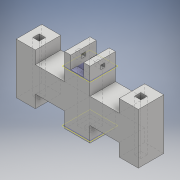
# Autodesk Inventor part: PRING_piston
Saved by Autodesk Inventor 2018 (Build 220112000, 112)
## iProperties
Created: 2026-07-07
Part Number: PRING_piston
Material: Generic
Document SubType Name: Modeling
Designer: neo
Density: 1 g/cm^3
Appearance: Default
Author: neo
Autodesk Inventor part; units mm, degrees
ref_plane "YZ Plane" through (0, 0, 0) normal (1, 0, 0) x (0, 1, 0)
ref_plane "XZ Plane" through (0, 0, 0) normal (0, 1, 0) x (-1, 0, 0)
ref_plane "XY Plane" through (0, 0, 0) normal (0, 0, 1) x (1, 0, 0)
sketch "Sketch1" plane through (0, 0, 0) normal (0, 1, 0) x (-1, 0, 0)
  line L0 (41.98, 54.6032) -> (41.98, -104.2857) construction
  line L1 (-38.02, 54.6032) -> (-38.02, -101.9048) construction
  line L2 (49.98, -31.1313) -> (-46.02, -31.1313)
  line L3 (-46.02, -31.1313) -> (-46.02, -71.1313)
  line L4 (-46.02, -71.1313) -> (49.98, -71.1313)
  line L5 (49.98, -71.1313) -> (49.98, -31.1313)
  line L6 (1.98, 80.3555) -> (1.98, -108.9591)
  point P0 (0, 0)
  dimension "d0" = 80
  dimension "d1" = 8
  dimension "d2" = 40
  constraints: 14 end point, 3 vertical, 2 parallel, 1 horizontal, 1 perpendicular, 2 other
  measures "d0" distance between parallel lines of L1 L0
  measures "d1" distance between parallel lines of L0 L5
  measures "d2" distance of L4.end L2.start
extrude "Extrusion1" add sketch "Sketch1" along normal mid plane 20
sketch "Sketch2" plane through (46.02, 10, -71.1313) normal (0, 0, -1) x (-1, 0, 0)
  circle A0 centre (88, -10) radius 2.5 construction
  circle A1 centre (8, -10) radius 2.5 construction
  line L0 (10.5, -7.5) -> (5.5, -7.5)
  line L1 (5.5, -7.5) -> (5.5, -12.5)
  line L2 (5.5, -12.5) -> (10.5, -12.5)
  line L3 (10.5, -12.5) -> (10.5, -7.5)
  line L4 (85.5, -7.5) -> (90.5, -7.5)
  line L5 (90.5, -7.5) -> (90.5, -12.5)
  line L6 (90.5, -12.5) -> (85.5, -12.5)
  line L7 (85.5, -12.5) -> (85.5, -7.5)
  point P0 (46.02, -10)
  point P1 (88, -10)
  point P2 (8, -10)
  dimension "d5" = 5
  dimension "d6" = 5
  constraints: 16 end point, 8 tangent, 4 parallel, 2 centre point, 2 coincident, 2 horizontal, 2 perpendicular
  measures "d5" diameter of A0
  measures "d6" diameter of A1
extrude "Extrusion2" cut sketch "Sketch2" against normal through all
sketch "Sketch3" plane through (0, 10, 0) normal (0, 1, 0) x (1, 0, 0)
  line L0 (-49.98, 31.1313) -> (46.02, 31.1313) construction
  line L1 (46.02, 31.1313) -> (46.02, 71.1313) construction
  line L2 (46.02, 71.1313) -> (-49.98, 71.1313) construction
  line L3 (-49.98, 71.1313) -> (-49.98, 31.1313) construction
  line L4 (-34.98, 79.1313) -> (31.02, 79.1313)
  line L5 (31.02, 79.1313) -> (31.02, 61.1313)
  line L6 (31.02, 61.1313) -> (-34.98, 61.1313)
  line L7 (-34.98, 61.1313) -> (-34.98, 79.1313)
  line L8 (46.02, 31.1313) -> (-49.98, 31.1313) construction
  line L9 (-1.98, 31.1313) -> (-1.98, 128.9069) construction
  line L10 (-41.98, -54.6032) -> (-41.98, 104.2857) construction
  line L11 (-34.98, 23.1313) -> (31.02, 23.1313)
  line L12 (31.02, 23.1313) -> (31.02, 41.1313)
  line L13 (31.02, 41.1313) -> (-34.98, 41.1313)
  line L14 (-34.98, 41.1313) -> (-34.98, 23.1313)
  point P0 (0, 0)
  dimension "d9" = 7
  dimension "d10" = 10
  dimension "d11" = 18
  dimension "d14" = 10
  dimension "d15" = 18
  constraints: 18 end point, 4 parallel, 2 horizontal, 2 perpendicular, 1 collinear, 1 midpoint, 1 vertical, 2 other
  measures "d9" distance between parallel lines of L10 L7
  measures "d10" distance between parallel lines of L6 L2
  measures "d11" distance of L6.end L4.start
  measures "d14" distance between parallel lines of L13 L8
  measures "d15" distance of L13.end L11.start
extrude "Extrusion3" cut sketch "Sketch3" against normal through all
sketch "Sketch4" plane through (31.02, 10, -61.1313) normal (0, 0, -1) x (-1, 0, 0)
  line L0 (31.02, -10) -> (61.64, -10) construction
  line L1 (43, 0) -> (23, 0)
  line L2 (23, 0) -> (23, -20)
  line L3 (23, -20) -> (43, -20)
  line L4 (43, -20) -> (43, 0)
  line L5 (66, -20) -> (0, -20) construction
  line L6 (66, 0) -> (66, -20) construction
  line L7 (0, 0) -> (66, 0) construction
  line L8 (0, 0) -> (0, -20) construction
  line L9 (66, -20) -> (0, -20) construction
  line L10 (33, -20) -> (33, -66.7058) construction
  line L11 (66, -10) -> (82.2472, -10) construction
  dimension "d16" = 20
  constraints: 14 end point, 2 midpoint, 2 parallel, 2 perpendicular, 1 collinear, 1 vertical, 2 other
  measures "d16" distance of L1.start L1.end
extrude "Extrusion4" add sketch "Sketch4" along normal blind 12 and the other way blind 40.5
ref_plane "Work Plane1" through (31.02, 10, -71.1313) normal (0, 0, -1) x (-1, 0, 0)
sketch "Sketch5" plane through (31.02, 10, -71.1313) normal (0, 0, -1) x (-1, 0, 0)
  line L0 (43, 0) -> (23, 0) construction
  line L1 (23, 0) -> (23, -20) construction
  line L2 (23, -20) -> (43, -20) construction
  line L3 (43, -20) -> (43, 0) construction
  line L4 (38.1, -4.9) -> (27.9, -4.9)
  line L5 (27.9, -4.9) -> (27.9, -15.1)
  line L6 (27.9, -15.1) -> (38.1, -15.1)
  line L7 (38.1, -15.1) -> (38.1, -4.9)
  line L8 (43, 0) -> (23, 0) construction
  line L9 (33, 0) -> (33, -20) construction
  line L10 (43, -20) -> (43, 0) construction
  line L11 (43, -10) -> (23, -10) construction
  line L12 (23, 0) -> (23, -20) construction
  point P0 (31.02, -10)
  dimension "d28" = 10.2
  constraints: 12 end point, 4 midpoint, 2 parallel, 2 perpendicular, 1 horizontal, 2 other
  measures "d28" distance of L6.end L4.start
extrude "Extrusion5" cut sketch "Sketch5" against normal through all
ref_plane "Work Plane2" through (31.02, 10, -30.6313) normal (0, 0, -1) x (-1, 0, 0)
sketch "Sketch6" plane through (31.02, 10, -20.6313) normal (0, 0, 1) x (1, 0, 0)
  line L0 (-38.1, -25.1) -> (-27.9, -25.1)
  line L1 (-27.9, -25.1) -> (-27.9, 5.1)
  line L2 (-27.9, 5.1) -> (-38.1, 5.1)
  line L3 (-38.1, 5.1) -> (-38.1, -25.1)
  line L4 (-38.1, -4.9) -> (-27.9, -4.9) construction
  line L5 (-38.1, -15.1) -> (-38.1, -4.9) construction
  line L6 (-27.9, -15.1) -> (-38.1, -15.1) construction
  line L7 (-27.9, -4.9) -> (-27.9, -15.1) construction
  line L8 (-38.1, -15.1) -> (-38.1, -4.9) construction
  line L9 (-27.9, -4.9) -> (-27.9, -15.1) construction
  point P0 (-31.02, -10)
  dimension "d29" = 10
  dimension "d30" = 10
  constraints: 8 end point, 2 collinear, 2 parallel, 1 horizontal, 1 perpendicular
  measures "d29" distance between parallel lines of L0 L6
  measures "d30" distance between parallel lines of L2 L4
extrude "Extrusion6" cut sketch "Sketch6" against normal up to surface (10 mm away)
sketch "Sketch7" plane through (-11.98, -10, -41.1313) normal (-1, 0, 0) x (0, 0, 1)
  line L0 (10.5, -4) -> (10.5, 24) construction
  line L1 (0, 0) -> (0, 20) construction
  line L2 (20.5, 0) -> (0, 0) construction
  line L3 (20.5, 20) -> (20.5, 0) construction
  line L4 (0, 20) -> (20.5, 20) construction
  line L5 (20.5, 0) -> (20.5, 20) construction
  line L6 (20.5, 10) -> (1.9837, 10) construction
  line L7 (10.5, 0) -> (20.5, 0) construction
  line L8 (15.5, 0) -> (15.5, 20) construction
  line L9 (0, 20) -> (20.5, 20) construction
  circle A0 centre (15.5, 10) radius 1.5 construction
  line L10 (14, 8.5) -> (17, 8.5)
  line L11 (17, 8.5) -> (17, 11.5)
  line L12 (17, 11.5) -> (14, 11.5)
  line L13 (14, 11.5) -> (14, 8.5)
  point P0 (41.1313, 10)
  dimension "d31" = 3
  constraints: 12 end point, 4 tangent, 3 midpoint, 2 horizontal, 2 parallel, 1 centre point, 1 perpendicular, 1 point on line, 1 vertical
  measures "d31" diameter of A0
extrude "Extrusion7" cut sketch "Sketch7" against normal through all
sketch "Sketch8" plane through (31.02, 10, -73.1313) normal (0, 0, -1) x (-1, 0, 0)
  line L0 (43, 0) -> (23, 0) construction
  line L1 (23, 0) -> (23, -20) construction
  line L2 (23, -20) -> (43, -20) construction
  line L3 (43, -20) -> (43, 0) construction
  line L4 (43, -10) -> (23, -10) construction
  line L5 (23, 0) -> (23, -20) construction
  line L6 (23, -20) -> (43, -20) construction
  line L7 (33, -20) -> (33, 0) construction
  circle A0 centre (33, -10) radius 2 construction
  line L8 (35, -12) -> (31, -12)
  line L9 (31, -12) -> (31, -8)
  line L10 (31, -8) -> (35, -8)
  line L11 (35, -8) -> (35, -12)
  point P0 (31.02, -10)
  dimension "d34" = 4
  constraints: 12 end point, 5 midpoint, 3 tangent, 2 parallel, 1 centre point, 1 horizontal, 1 perpendicular
  measures "d34" diameter of A0
extrude "Extrusion8" cut sketch "Sketch8" against normal blind 20
equation "\"d6\" = d5"
body "Solid1"
